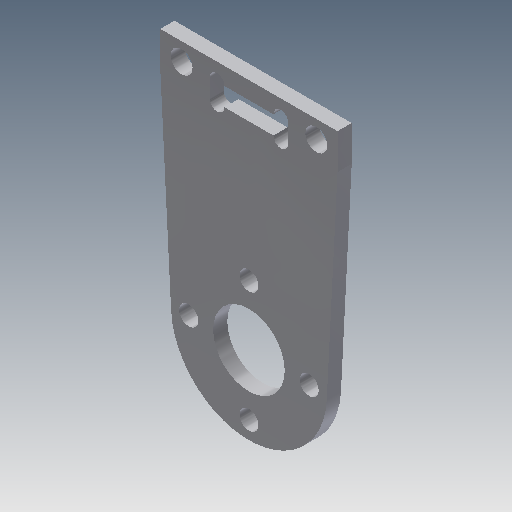
# Autodesk Inventor part: 付け根ロール_サブフレーム_1_1
Saved by Autodesk Inventor 2017.3 (Build 213256000, 256)
## iProperties
Created: 2016-05-01
Part Number: 付け根ロール_サブフレーム_1_1
Material: アルミニウム 2014-T4
Document SubType Name: Modeling
Designer: hiroaki
Density: 2.8 g/cm^3
Appearance: サテン
Mass: 3.48692 g
Surface Area: 22.678 cm^2
Volume: 1.24533 cm^3
Author: hiroaki
Autodesk Inventor part; units mm, degrees
ref_plane "YZ Plane" through (0, 0, 0) normal (1, 0, 0) x (0, 1, 0)
ref_plane "XZ Plane" through (0, 0, 0) normal (0, 1, 0) x (-1, 0, 0)
ref_plane "XY Plane" through (0, 0, 0) normal (0, 0, 1) x (1, 0, 0)
derived "付け根ロール_基礎_2.ipt"
sketch "スケッチ1" plane through (0, 0, 0) normal (0, 0, 1) x (1, 0, 0)
  circle A0 centre (0, 0) radius 5.05
  circle A1 centre (0, 8.5) radius 1.35
  circle A2 centre (-8.5, 0) radius 1.35
  circle A3 centre (0, -8.5) radius 1.35
  circle A4 centre (8.5, 0) radius 1.35
  line L0 (-12.5, 28) -> (-10.9846, -0.5824)
  line L1 (-12.5, 28) -> (-12.5, 30.5)
  line L2 (12.5, 28) -> (10.9846, -0.5824)
  arc A5 (-10.9846, -0.5824) -> (10.9846, -0.5824) centre (0, 0) ccw
  line L3 (12.5, 30.5) -> (-12.5, 30.5) construction
  line L4 (-12.5, 30.5) -> (-12.5, 28) construction
  line L5 (-12.5, 28) -> (12.5, 28) construction
  line L6 (-29.05, 12) -> (29.25, 12) construction
  line L7 (29.25, 12) -> (29.25, -11) construction
  line L8 (29.25, -11) -> (-29.05, -11) construction
  line L9 (-29.05, -11) -> (-29.05, 12) construction
  circle A6 centre (0, 0) radius 31.6159 construction
  circle A7 centre (-9.5, 30.5) radius 1.55
  line L10 (-12.5, 30.5) -> (-12.5, 33)
  line L11 (-12.5, 33) -> (12.5, 33)
  line L12 (12.5, 33) -> (12.5, 30.5)
  line L13 (12.5, 30.5) -> (12.5, 28) construction
  line L14 (12.5, 30.5) -> (12.5, 28)
  line L15 (-5.5, 30.5) -> (5.5, 30.5) construction
  line L16 (5.5, 30.5) -> (5.5, 28) construction
  line L17 (5.5, 28) -> (-5.5, 28) construction
  line L18 (-5.5, 28) -> (-5.5, 30.5) construction
  circle A8 centre (9.5, 30.5) radius 1.55
  line L19 (0, 0) -> (0, 5.5002) construction
  line L20 (5.55, 27.95) -> (5.55, 30.55) construction
  line L21 (5.55, 30.55) -> (-5.55, 30.55) construction
  line L22 (-5.55, 30.55) -> (-5.55, 27.95) construction
  line L23 (-5.55, 27.95) -> (5.55, 27.95) construction
  circle A9 centre (-4.5, 30.55) radius 1.05 construction
  line L24 (-5.55, 30.55) -> (-5.55, 27.95)
  arc A10 (-3.45, 30.55) -> (-5.55, 30.55) centre (-4.5, 30.55) ccw
  line L25 (-3.45, 30.55) -> (3.45, 30.55)
  arc A11 (-5.55, 27.95) -> (-3.45, 27.95) centre (-4.5, 27.95) ccw
  line L26 (5.55, 29.25) -> (-5.55, 29.25) construction
  line L27 (-3.45, 27.95) -> (3.45, 27.95)
  line L28 (5.55, 30.55) -> (5.55, 27.95)
  arc A12 (5.55, 30.55) -> (3.45, 30.55) centre (4.5, 30.55) ccw
  arc A13 (3.45, 27.95) -> (5.55, 27.95) centre (4.5, 27.95) ccw
  line L29 (-5.55, 30.55) -> (-4.5, 30.55) construction
  circle A14 centre (-9.5, 30.5) radius 3 construction
  point P0 (0, 30.5)
  point P1 (-12.5, 29.25)
  point P2 (0, 30.5)
  point P3 (0, 30.5)
  point P4 (0, 33)
extrude "押し出し1" add sketch "スケッチ1" along normal blind 2
sketch "スケッチ3" plane through (0, 0, 0) normal (0, 0, -1) x (-1, 0, 0)
  circle A0 centre (0, 0) radius 5.05 projected
  line L0 (-3.45, 30.55) -> (3.45, 30.55) projected
  line L1 (3.45, 27.95) -> (-3.45, 27.95) projected
  circle A1 centre (0, 8.5) radius 1.35 projected
  line L2 (-10.9846, -0.5824) -> (-12.5, 28) projected
  arc A2 (-10.9846, -0.5824) -> (10.9846, -0.5824) centre (0, 0) ccw projected
  line L3 (-10.3381, 25) -> (-9.3222, 5.8392)
  circle A3 centre (0, 0) radius 11 construction
  arc A4 (-1.5, 10.8972) -> (-9.3222, 5.8392) centre (0, 0) ccw
  line L4 (-10.3381, 25) -> (-1.5, 25)
  line L5 (-1.5, 25) -> (-1.5, 10.8972)
  line L6 (-4.1931, 28.8141) -> (4.1798, 28.8141)
  line L7 (4.1798, 28.8141) -> (4.1798, 28)
  line L8 (4.1798, 28) -> (-4.1931, 28)
  line L9 (-4.1931, 28) -> (-4.1931, 28.8141)
  line L10 (0, 30.55) -> (0, 8.5) construction
  line L11 (10.3381, 25) -> (9.3222, 5.8392)
  arc A5 (9.3222, 5.8392) -> (1.5, 10.8972) centre (0, 0) ccw
  line L12 (10.3381, 25) -> (1.5, 25)
  line L13 (1.5, 25) -> (1.5, 10.8972)
  dimension "d3" = 1.5
  dimension "d4" = 2
  dimension "d5" = 0.05
  dimension "d6" = 3
  constraints: 22 end point, 4 point on circle, 4 symmetric about line, 3 centre point, 3 parallel, 2 coincident, 2 concentric, 2 horizontal, 2 vertical, 1 midpoint, 1 perpendicular, 1 other
  measures "d3" distance from line of L10.end L5
  measures "d4" distance between parallel lines of L2 L3
  measures "d5" distance between parallel lines of L1 L8
  measures "d6" distance between parallel lines of L4 L8
extrude "押し出し2" cut sketch "スケッチ3" against normal blind 1.5 contours L4 L5 A4 L3 | L11 A5 L13 L12
fillet "フィレット1" radius 1.05 8 edges at (9.3222, 5.8392, 0.75) (1.5, 10.8972, 0.75) (10.3381, 25, 0.75) (-1.5, 10.8972, 0.75) (-9.3222, 5.8392, 0.75) (-1.5, 25, 0.75) (1.5, 25, 0.75) (-10.3381, 25, 0.75)
